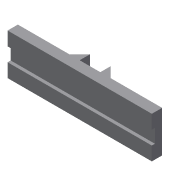
# Autodesk Inventor part: Tank Tread link A
Saved by Autodesk Inventor 2015 (Build 190159000, 159)
## iProperties
Created: 2015-03-14
Part Number: Tank Tread link A
Material: Generic
Document SubType Name: Modeling
Designer: james_000
Density: 1 g/cm^3
Appearance: Default
Author: james_000
Autodesk Inventor part; units mm, degrees
ref_plane "YZ Plane" through (0, 0, 0) normal (1, 0, 0) x (0, 1, 0)
ref_plane "XZ Plane" through (0, 0, 0) normal (0, 1, 0) x (-1, 0, 0)
ref_plane "XY Plane" through (0, 0, 0) normal (0, 0, 1) x (1, 0, 0)
sketch "Sketch1" plane through (0, 0, 0) normal (0, 0, 1) x (1, 0, 0)
  line L0 (0, 0) -> (7, 0)
  line L1 (0, 0) -> (-7, 0)
  line L2 (-7, 0) -> (-7, 1)
  line L3 (7, 1) -> (7, 0)
  line L4 (-7, 1) -> (-2, 1)
  line L5 (2, 1) -> (7, 1)
  line L6 (-1, 2) -> (-2, 1)
  line L7 (1, 2) -> (2, 1)
  line L8 (-1, 2) -> (-1, 1)
  line L9 (-1, 1) -> (1, 1)
  line L10 (1, 1) -> (1, 2)
  dimension "d1" = 7
  dimension "d2" = 1
  dimension "d7" = 2
  dimension "d8" = 1
  dimension "d9" = 2
  constraints: 22 end point, 3 horizontal, 3 perpendicular, 2 point on line, 1 vertical
  measures "d1" distance of L0.start L1.end
  measures "d2" distance of L1.end L2.end
  measures "d7" distance of L6.start L7.start
  measures "d8" distance of L6.start L8.end
  measures "d9" distance of L8.end L9.end
extrude "Extrusion1" add sketch "Sketch1" along normal blind 4
sketch "Sketch2" plane through (-1, 1, 0) normal (1, 0, 0) x (0, 0, -1)
  line L0 (0, 0) -> (0, 1) projected
  line L1 (-4, 0) -> (-4, 1) projected
  circle A0 centre (-1, 0.5) radius 0.25
  circle A1 centre (-3, 0.5) radius 0.25
  point P0 (0, -1)
  dimension "d14" = 0.5
  dimension "d15" = 0.5
  constraints: 2 centre point
  measures "d14" diameter of A0
  measures "d15" diameter of A1
extrude "Extrusion2" add sketch "Sketch2" along normal blind 2 contours A0
sketch "Sketch3" plane through (-1, 1, 0) normal (1, 0, 0) x (0, 0, -1)
  line L0 (-4, 0) -> (-4, 1) projected
  circle A0 centre (-3, 0.5) radius 0.25
  point P0 (0, -1)
  dimension "d19" = 0.5
  constraints: 1 centre point
  measures "d19" diameter of A0
extrude "Extrusion3" add sketch "Sketch3" along normal blind 2
sketch "Sketch4" plane through (7, 0, 0) normal (1, 0, 0) x (0, 0, -1)
  line L0 (0, 0) -> (-1.3333, 0)
  line L1 (-1.3333, 0) -> (-1.3333, 0.3)
  line L2 (-1.3333, 0.3) -> (-2.6667, 0.3)
  line L3 (-2.6667, 0.3) -> (-2.6667, 0)
  point P0 (-4, 0)
  dimension "d22" = 1.3333
  dimension "d23" = 1.3333
  dimension "d24" = 0.3
  constraints: 8 end point, 2 perpendicular
  measures "d22" distance of point (-4, 0) L3.end
  measures "d23" distance of L0.start L0.end
  measures "d24" distance of L0.end L1.end
split body "Split1" sketch "Sketch4" result one side removed curves L0 L1 L2 L3 removed pieces at (-2.3333, 0.1, 1.7778)
body "Solid1"
